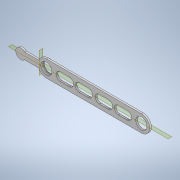
# Autodesk Inventor part: p1
Saved by Autodesk Inventor 2022 (Build 260153000, 153)
## iProperties
Created: 2022-03-17
Part Number: p1
Material: Generic
Document SubType Name: Modeling
Designer: br4ch
Density: 1 g/cm^3
Appearance: Default
Author: br4ch
Autodesk Inventor part; units mm, degrees
ref_plane "YZ Plane" through (0, 0, 0) normal (1, 0, 0) x (0, 1, 0)
ref_plane "XZ Plane" through (0, 0, 0) normal (0, 1, 0) x (-1, 0, 0)
ref_plane "XY Plane" through (0, 0, 0) normal (0, 0, 1) x (1, 0, 0)
sketch "Sketch2" plane through (0, 0, 0) normal (0, 0, 1) x (1, 0, 0)
  line L0 (-108, -20.3137) -> (62, -20.3137) construction
  line L1 (-108, -35.3137) -> (62, -35.3137)
  line L2 (62, -5.3137) -> (-108, -5.3137)
  arc A0 (-108, -5.3137) -> (-108, -35.3137) centre (-108, -20.3137) ccw
  arc A1 (62, -35.3137) -> (62, -5.3137) centre (62, -20.3137) ccw
  circle A2 centre (-108, -20.3137) radius 10
  circle A3 centre (62, -20.3137) radius 10
  line L3 (-83, -20.3137) -> (-67, -20.3137) construction
  line L4 (-83, -27.8137) -> (-67, -27.8137)
  line L5 (-67, -12.8137) -> (-83, -12.8137)
  arc A4 (-83, -12.8137) -> (-83, -27.8137) centre (-83, -20.3137) ccw
  arc A5 (-67, -27.8137) -> (-67, -12.8137) centre (-67, -20.3137) ccw
  line L6 (-23, -46) -> (-23, 6) construction
  arc A6 (-33, -27.8137) -> (-33, -12.8137) centre (-33, -20.3137) ccw
  line L7 (-49, -20.3137) -> (-33, -20.3137) construction
  line L8 (-49, -27.8137) -> (-33, -27.8137)
  line L9 (-33, -12.8137) -> (-49, -12.8137)
  arc A7 (-49, -12.8137) -> (-49, -27.8137) centre (-49, -20.3137) ccw
  line L10 (37, -20.3137) -> (21, -20.3137) construction
  line L11 (37, -27.8137) -> (21, -27.8137)
  line L12 (21, -12.8137) -> (37, -12.8137)
  arc A8 (37, -27.8137) -> (37, -12.8137) centre (37, -20.3137) ccw
  arc A9 (21, -12.8137) -> (21, -27.8137) centre (21, -20.3137) ccw
  arc A10 (-13, -12.8137) -> (-13, -27.8137) centre (-13, -20.3137) ccw
  line L13 (3, -20.3137) -> (-13, -20.3137) construction
  line L14 (3, -27.8137) -> (-13, -27.8137)
  line L15 (-13, -12.8137) -> (3, -12.8137)
  arc A11 (3, -27.8137) -> (3, -12.8137) centre (3, -20.3137) ccw
  line L16 (-121.6954, -14.1952) -> (-147.279, -14.1952)
  line L17 (-121.6954, -26.4323) -> (-147.279, -26.4323)
  circle A12 centre (-154, -20.3137) radius 9.0889
  circle A13 centre (-108, -20.3137) radius 12.5
  line L18 (-119.5282, -20.3137) -> (-121.5282, -20.3137)
  point P0 (0, 0)
  point P1 (-23, -20.3137)
  point P2 (-75, -20.3137)
  point P3 (-41, -20.3137)
  point P4 (29, -20.3137)
  point P5 (-5, -20.3137)
  point P6 (-120.5, -20.3137)
  dimension "d51" = 25
  dimension "d27" = 170
  dimension "d28" = 30
  dimension "d29" = 20
  dimension "d30" = 20
  dimension "d31" = 16
  dimension "d32" = 15
  dimension "d43" = 34
  dimension "d48" = 41
  dimension "d57" = 2
  constraints: 48 end point, 21 point on circle, 16 symmetric about line, 12 centre point, 8 tangent, 5 horizontal, 4 point on line, 3 coincident, 2 midpoint, 2 parallel, 1 horizontal alignment, 1 vertical, 21 other
  measures "d27" distance of L0.start L0.end
  measures "d28" diameter of A1
  measures "d29" diameter of A2
  measures "d30" diameter of A3
  measures "d31" distance of L3.start L3.end
  measures "d32" diameter of A5
  measures "d43" distance of L3.end L7.end
  measures "d48" distance of L3.end L0.start
  measures "d57" distance of L18.start L18.end
extrude "Extrusion2" add sketch "Sketch2" along normal blind 3 contours A0 L2 A1 L1 | L17 A12 L16 A0 | A12 | A13
extrude "Extrusion3" add sketch "Sketch2" against normal blind 3 contours A13
ref_plane "Work Plane1" through (-119.5282, -20.3137, 0) normal (0, -1, 0) x (-1, 0, 0)
sketch "Sketch4" plane through (-108, -20.3137, -3) normal (0, 0, -1) x (-1, 0, 0)
  line L0 (11.5282, 0) -> (13.5282, 0) projected
  circle A0 centre (0, 0) radius 12.5 projected
  point P0 (-108, 20.3137)
  point P1 (12.5, 0)
  constraints: 1 horizontal alignment, 1 point on line, 1 other
ref_plane "Work Plane2" through (-120.5, -20.3137, -3) normal (-1, 0, 0) x (0, -1, 0)
sketch "Sketch5" plane through (-120.5, -20.3137, -3) normal (-1, 0, 0) x (0, -1, 0)
  line L0 (9.0889, 3) -> (-9.0889, 3) projected
  line L1 (-12.5, 0) -> (12.5, 0) projected
  line L2 (0, -1.2) -> (0, 7.2) projected
  line L3 (15, 3) -> (-15, 3) projected
  line L4 (0, 3) -> (0, 0)
  line L5 (10, 0) -> (-10, 0) projected
  line L6 (0, 3) -> (0, 0)
  circle A0 centre (0, 1.5) radius 0.25
  point P0 (-20.3137, 3)
  point P1 (-6.1186, 3)
  point P2 (6.1186, 3)
  dimension "d63" = 0.5
  constraints: 4 end point, 3 midpoint, 2 coincident, 1 centre point, 1 collinear
  measures "d63" diameter of A0
extrude "Extrusion5" cut sketch "Sketch5" against normal up to surface round surface about axis through (-108, -20.3137, 0) along (0, 0, 1) radius 10 far side no
pattern_circular "Circular Pattern1" count 3 over 360 about axis through (-108, -20.3137, 0) along (0, 0, -1) of "Extrusion5"
body "Solid2"
